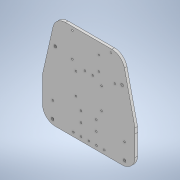
# Autodesk Inventor part: Base
Saved by Autodesk Inventor 2020 (Build 240168000, 168)
## iProperties
Created: 2020-11-22
Part Number: Base
Material: Generic
Document SubType Name: Modeling
Designer: michelin
Density: 1 g/cm^3
Appearance: Default
Author: michelin
Autodesk Inventor part; units mm, degrees
ref_plane "YZ Plane" through (0, 0, 0) normal (1, 0, 0) x (0, 1, 0)
ref_plane "XZ Plane" through (0, 0, 0) normal (0, 1, 0) x (-1, 0, 0)
ref_plane "XY Plane" through (0, 0, 0) normal (0, 0, 1) x (1, 0, 0)
sketch "Base" plane through (0, 0, 0) normal (0, 0, 1) x (1, 0, 0)
  line L0 (54.795, 156.8823) -> (-53.4125, 156.8823)
  line L1 (-53.4125, 156.8823) -> (-53.4125, 210.2985)
  line L2 (-53.4125, 210.2985) -> (54.795, 210.2985)
  line L3 (54.795, 210.2985) -> (54.795, 156.8823)
  circle A0 centre (50.5227, 159.5184) radius 1.5621
  circle A1 centre (50.5227, 159.5184) radius 1.5621
  circle A2 centre (19.522, 164.3969) radius 1.5621
  circle A3 centre (19.522, 164.3969) radius 1.5621
  circle A4 centre (-32.1035, 159.5184) radius 1.5621
  circle A5 centre (-32.1035, 159.5184) radius 1.5621
  circle A6 centre (19.522, 192.4131) radius 1.3153
  circle A7 centre (43.0297, 207.8546) radius 1.5621
  circle A8 centre (43.0297, 207.8546) radius 1.5621
  circle A9 centre (-32.1035, 207.8546) radius 1.5621
  circle A10 centre (-32.1035, 207.8546) radius 1.5621
  line L4 (-1.4408, 214.4401) -> (-65.4669, 214.4401)
  line L5 (-90.4669, 29.5677) -> (89.5331, 29.5677)
  line L6 (34.9232, 45.6333) -> (34.9232, 29.6333)
  line L7 (-35.0768, 29.6333) -> (-35.0768, 45.6333)
  line L8 (34.9232, 45.6333) -> (-35.0768, 45.6333)
  line L9 (-35.0768, 29.6333) -> (34.9232, 29.6333)
  circle A11 centre (29.9232, 37.6333) radius 1.5875
  circle A12 centre (14.9232, 37.6333) radius 1.5875
  circle A13 centre (-0.0768, 37.6333) radius 1.5875
  circle A14 centre (-0.0768, 37.6333) radius 1.5875
  circle A15 centre (-15.0768, 37.6333) radius 1.5875
  circle A16 centre (-30.0768, 37.6333) radius 1.5875
  line L10 (-10.0624, 153.9875) -> (-10.0624, 149.9875)
  line L11 (9.9376, 149.9875) -> (9.9376, 153.9875)
  line L12 (-10.0624, 149.9875) -> (-10.0624, 153.9875)
  line L13 (-10.0624, 153.9875) -> (9.9376, 153.9875)
  line L14 (9.9376, 153.9875) -> (9.9376, 149.9875)
  line L15 (9.9376, 149.9875) -> (-10.0624, 149.9875)
  circle A17 centre (-7.5624, 151.9875) radius 1.5875
  circle A18 centre (-7.5624, 151.9875) radius 1.5875
  circle A19 centre (7.4376, 151.9875) radius 1.5875
  circle A20 centre (7.4376, 151.9875) radius 1.5875
  circle A21 centre (-346.1506, -30.1346) radius 0.95
  circle A22 centre (-346.1506, -30.1346) radius 16
  circle A23 centre (-346.1506, -30.1346) radius 17.4
  circle A24 centre (-346.1506, -30.1346) radius 18.4
  circle A25 centre (-346.1506, -30.1346) radius 17
  line L16 (-335.9251, -43.7154) -> (-336.3078, -42.7916)
  line L17 (-335.9251, -43.7154) -> (-336.3078, -42.7916)
  line L18 (-344.1607, -46.0444) -> (-343.7781, -46.9682)
  line L19 (-343.7781, -46.9682) -> (-344.1607, -46.0444)
  line L20 (-359.7314, -40.3601) -> (-358.8075, -39.9775)
  line L21 (-359.7314, -40.3601) -> (-358.8075, -39.9775)
  line L22 (-362.0604, -32.1245) -> (-362.9842, -32.5072)
  line L23 (-362.9842, -32.5072) -> (-362.0604, -32.1245)
  line L24 (-343.7781, -13.301) -> (-344.1607, -14.2249)
  line L25 (-343.7781, -13.301) -> (-344.1607, -14.2249)
  line L26 (-336.3078, -17.4777) -> (-335.9251, -16.5538)
  line L27 (-335.9251, -16.5538) -> (-336.3078, -17.4777)
  line L28 (-0.4669, 29.5677) -> (-3.8896, 29.5677)
  circle A26 centre (-30.0768, 37.6333) radius 1.5875
  circle A27 centre (-30.0768, 37.6333) radius 1.5875
  line L29 (-90.4669, 29.5677) -> (-90.4669, 104.3985)
  line L30 (114.5331, -0.4323) -> (89.5331, -0.4323)
  line L31 (89.5331, 29.5677) -> (89.5331, 94.2566)
  line L32 (10.3338, -39.9759) -> (10.0469, -40.3854)
  arc A28 (6.6378, -33.8337) -> (10.0469, -40.3854) centre (14.6378, -33.8337) ccw
  line L33 (6.6378, -25.8337) -> (6.6378, -33.8337)
  line L34 (6.6378, -33.8337) -> (6.6378, -25.8337)
  arc A29 (14.6378, -17.8337) -> (6.6378, -25.8337) centre (14.6378, -25.8337) ccw
  line L35 (14.6378, -17.8337) -> (45.6378, -17.8337)
  arc A30 (53.6378, -25.8337) -> (45.6378, -17.8337) centre (45.6378, -25.8337) ccw
  line L36 (53.6378, -33.8337) -> (53.6378, -25.8337)
  line L37 (53.6378, -25.8336) -> (53.6378, -33.8337)
  arc A31 (45.6378, -41.8337) -> (53.6378, -33.8337) centre (45.6378, -33.8337) ccw
  arc A32 (14.6378, -17.8337) -> (6.6378, -25.8337) centre (14.6378, -25.8337) ccw
  arc A33 (6.6378, -33.8337) -> (14.6378, -41.8337) centre (14.6378, -33.8337) ccw
  arc A34 (45.6378, -41.8337) -> (53.6378, -33.8337) centre (45.6378, -33.8337) ccw
  arc A35 (53.6378, -25.8337) -> (45.6378, -17.8337) centre (45.6378, -25.8337) ccw
  line L38 (14.6378, -41.8337) -> (45.6378, -41.8337)
  line L39 (14.6378, -41.8337) -> (31.3301, -41.8337)
  line L40 (31.3301, -17.8337) -> (31.3301, -41.8337)
  line L41 (6.6378, -29.8337) -> (31.3301, -29.8337)
  line L42 (-50.1942, 121.7471) -> (-50.1942, 137.7471)
  line L43 (-50.1942, 137.7471) -> (49.8058, 137.7471)
  line L44 (-50.1942, 121.7471) -> (-50.1942, 105.7471)
  line L45 (-50.1942, 105.7471) -> (49.8058, 105.7471)
  line L46 (49.8058, 105.7471) -> (49.8058, 137.7471)
  line L47 (49.8058, 105.7471) -> (29.8058, 105.7471)
  line L48 (29.8058, 105.7471) -> (29.8058, 95.7471)
  line L49 (29.8058, 95.7471) -> (19.8058, 95.7471)
  line L50 (19.8058, 95.7471) -> (19.8058, 105.7471)
  line L51 (-50.1942, 105.7471) -> (-30.1942, 105.7471)
  line L52 (-30.1942, 105.7471) -> (-30.1942, 95.7471)
  line L53 (-30.1942, 95.7471) -> (-20.1942, 95.7471)
  line L54 (-20.1942, 95.7471) -> (-20.1942, 105.7471)
  line L55 (49.8058, 137.7471) -> (29.8058, 137.7471)
  line L56 (29.8058, 137.7471) -> (29.8058, 147.7471)
  line L57 (29.8058, 147.7471) -> (19.8058, 147.7471)
  line L58 (19.8058, 147.7471) -> (19.8058, 137.7471)
  line L59 (-50.1942, 137.7471) -> (-30.1942, 137.7471)
  line L60 (-30.1942, 137.7471) -> (-30.1942, 147.7471)
  line L61 (-30.1942, 147.7471) -> (-20.1942, 147.7471)
  line L62 (-20.1942, 147.7471) -> (-20.1942, 137.7471)
  line L63 (-30.1942, 137.7471) -> (-25.1942, 137.7471)
  line L64 (-30.1942, 105.7471) -> (-25.1942, 105.7471)
  line L65 (-30.1942, 105.7471) -> (-25.1942, 105.7471)
  line L66 (19.8058, 137.7471) -> (24.8058, 137.7471)
  line L67 (19.8058, 105.7471) -> (24.8058, 105.7471)
  circle A36 centre (-25.1942, 142.7471) radius 1.5875
  circle A37 centre (24.8058, 142.7471) radius 1.5875
  circle A38 centre (-25.1942, 100.7471) radius 1.5875
  circle A39 centre (24.8058, 100.7471) radius 1.5875
  line L68 (-1.4408, 214.4401) -> (64.5331, 214.4401)
  line L69 (-65.4669, 214.4401) -> (-40.4669, 214.4401)
  line L70 (64.5331, 214.4401) -> (39.5331, 214.4401)
  line L71 (89.4944, 52.4566) -> (19.3944, 52.4566)
  line L72 (19.3944, 52.4566) -> (19.3944, 89.2566)
  line L73 (19.3944, 89.2566) -> (89.4944, 89.2566)
  line L74 (89.4944, 89.2566) -> (89.4944, 52.4566)
  line L75 (-20.2126, 89.3997) -> (-20.2126, 52.5997)
  line L76 (-20.2126, 52.5997) -> (-90.3126, 52.5997)
  line L77 (-90.3126, 52.5997) -> (-90.3126, 89.3997)
  line L78 (-90.3126, 89.3997) -> (-20.2126, 89.3997)
  line L79 (-20.2126, 89.3997) -> (-20.2126, 52.5997)
  line L80 (-20.2126, 52.5997) -> (-10.2126, 52.5997)
  line L81 (-10.2126, 52.5997) -> (-10.2126, 89.3997)
  line L82 (-10.2126, 89.3997) -> (-20.2126, 89.3997)
  circle A40 centre (-15.2126, 80.9997) radius 1.5875
  circle A41 centre (-15.2126, 60.9997) radius 1.5875
  line L83 (19.3944, 52.4566) -> (9.3944, 52.4566)
  line L84 (9.3944, 52.4566) -> (9.3944, 89.2566)
  line L85 (9.3944, 89.2566) -> (19.3944, 89.2566)
  circle A42 centre (14.3944, 80.8566) radius 1.5875
  circle A43 centre (14.3944, 60.8566) radius 1.5875
  line L86 (-90.3126, 89.3997) -> (-90.3126, 94.3997)
  line L87 (-90.3126, 94.3997) -> (-10.2126, 94.3997)
  line L88 (-10.2126, 94.3997) -> (-10.2126, 89.3997)
  line L89 (-10.2126, 52.5997) -> (-10.2126, 47.5997)
  line L90 (-10.2126, 47.5997) -> (-90.3126, 47.5997)
  line L91 (-90.3126, 47.5997) -> (-90.3126, 52.5997)
  line L92 (9.3944, 52.4566) -> (9.3944, 47.4566)
  line L93 (9.3944, 47.4566) -> (89.4566, 47.4566)
  line L94 (89.4566, 47.4566) -> (89.4944, 52.4566)
  line L95 (89.4944, 89.2566) -> (89.4944, 94.2566)
  line L96 (89.4944, 94.2566) -> (9.3944, 94.2566)
  line L97 (9.3944, 94.2566) -> (9.3944, 89.2566)
  line L98 (-90.3126, 94.3997) -> (-90.4669, 104.3985)
  line L99 (-90.4669, 104.3985) -> (-65.4669, 214.4401)
  line L100 (89.4944, 94.2566) -> (89.4944, 104.2566)
  line L101 (89.4944, 104.2566) -> (64.5331, 214.4401)
  line L102 (-90.4669, 29.5677) -> (-70.4669, 29.5677)
  line L103 (89.5331, 29.5677) -> (69.5331, 29.5677)
  line L104 (-90.3126, 94.3997) -> (-65.3126, 94.3997)
  line L105 (89.5331, 94.2566) -> (64.5331, 94.2566)
  circle A44 centre (-65.3126, 164.3997) radius 2.5
  circle A45 centre (64.5331, 164.2566) radius 2.5
  circle A46 centre (69.5331, 39.5677) radius 2.5
  circle A47 centre (-70.4669, 39.5677) radius 2.5
  line L106 (-20.2126, 52.5997) -> (-70.2126, 52.5997)
  line L107 (-70.2126, 52.5997) -> (-70.2126, 70.9997)
  line L108 (19.3944, 52.4566) -> (69.3944, 52.4566)
  line L109 (69.3944, 52.4566) -> (69.3944, 70.8566)
  circle A48 centre (-70.2126, 70.9997) radius 1.5875
  circle A49 centre (69.3944, 70.8566) radius 1.5875
  point P0 (-0.0768, 37.6333)
  point P1 (-0.0624, 151.9875)
  dimension "d72" = 50
  dimension "d73" = 18.4
  dimension "d74" = 50
  dimension "d75" = 18.4
  dimension "d76" = 3.175
  dimension "d77" = 3.175
  constraints: 220 end point, 50 centre point, 32 point on line, 25 perpendicular, 19 point on circle, 18 coincident, 9 collinear, 8 parallel, 7 horizontal, 4 vertical, 3 concentric, 3 midpoint
  measures "d72" distance of L79.end L106.end
  measures "d73" distance of L106.end L107.end
  measures "d74" distance of L83.start L108.end
  measures "d75" distance of L108.end L109.end
  measures "d76" diameter of A48
  measures "d77" diameter of A49
extrude "Extrusion1" add sketch "Base" along normal blind 5 contours L0 L1 L2 L3 | L95 L73 L85 L97 L96 | L68 L101 L100 L105 L31 L5 L29 L99 L4 | L74 L71 L72 L73 | L72 L83 L84 L85 | L94 L93 L92 L83 L71 | L6 L9 L7 L8 | L13 L11 L15 L10 | L42 L43 L46 L45 L44 | L60 L61 L62 L43 | L45 L54 L53 L52 | L58 L57 L56 L43 | L45 L48 L49 L50 | L82 L81 L80 L75 | L75 L76 L77 L78 | L78 L86 L87 L88 L82 | L80 L89 L90 L91 L76
fillet "Fillet1" radius 25 4 edges at (89.5331, 29.5677, 2.5) (64.5331, 214.4401, 2.5) (-65.4669, 214.4401, 2.5) (-90.4669, 29.5677, 2.5)
body "Solid1"
